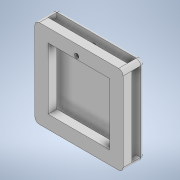
# Autodesk Inventor part: the structure
Saved by Autodesk Inventor 2022 (Build 260153000, 153)
## iProperties
Created: 2021-07-07
Part Number: the structure
Material: Generic
Document SubType Name: Modeling
Designer: fanam
Density: 1 g/cm^3
Appearance: Default
Author: fanam
Autodesk Inventor part; units mm, degrees
ref_plane "YZ Plane" through (0, 0, 0) normal (1, 0, 0) x (0, 1, 0)
ref_plane "XZ Plane" through (0, 0, 0) normal (0, 1, 0) x (-1, 0, 0)
ref_plane "XY Plane" through (0, 0, 0) normal (0, 0, 1) x (1, 0, 0)
sketch "Sketch1" plane through (0, 0, 0) normal (0, 0, 1) x (1, 0, 0)
  line L0 (0, 0) -> (1000, 0)
  line L1 (1000, 0) -> (1000, 1000)
  line L2 (1000, 1000) -> (0, 1000)
  line L3 (0, 1000) -> (0, 0)
  dimension "d0" = 1000
  dimension "d1" = 1000
  constraints: 8 end point, 2 parallel, 1 horizontal, 1 perpendicular
  measures "d0" distance of L2.end L1.end
  measures "d1" distance of L1.end L0.end
extrude "Extrusion1" add sketch "Sketch1" along normal blind 250
sketch "Sketch6" plane through (0, 1000, 0) normal (0, 1, 0) x (1, 0, 0)
  line L0 (50, -150) -> (950, -150)
  line L1 (950, -150) -> (950, -50)
  line L2 (950, -50) -> (50, -50)
  line L3 (50, -50) -> (50, -150)
  line L4 (1000, 0) -> (0, 0) projected
  line L5 (1000, 0) -> (1000, -250) projected
  dimension "d14" = 900
  dimension "d15" = 100
  dimension "d16" = 50
  dimension "d17" = 50
  constraints: 8 end point, 2 parallel, 1 horizontal, 1 perpendicular
  measures "d14" distance of L0.start L0.end
  measures "d15" distance of L0.end L1.end
  measures "d16" distance between parallel lines of L2 L4
  measures "d17" distance between parallel lines of L5 L1
extrude "Extrusion3" cut sketch "Sketch6" against normal blind 1000
sketch "Sketch7" plane through (1000, 0, 0) normal (1, 0, 0) x (0, 0, -1)
  line L0 (-150, 950) -> (-50, 950)
  line L1 (-50, 950) -> (-50, 50)
  line L2 (-50, 50) -> (-150, 50)
  line L3 (-150, 50) -> (-150, 950)
  line L4 (0, 0) -> (0, 1000) projected
  line L5 (0, 0) -> (-250, 0) projected
  dimension "d20" = 900
  dimension "d21" = 100
  dimension "d22" = 50
  dimension "d23" = 50
  constraints: 8 end point, 2 parallel, 1 horizontal, 1 perpendicular
  measures "d20" distance of L2.end L0.start
  measures "d21" distance of L1.end L2.end
  measures "d22" distance between parallel lines of L4 L1
  measures "d23" distance between parallel lines of L5 L2
extrude "Extrusion4" cut sketch "Sketch7" against normal blind 1000
sketch "Sketch8" plane through (0, 0, 250) normal (0, 0, 1) x (1, 0, 0)
  line L0 (150, 150) -> (850, 150)
  line L1 (850, 150) -> (850, 850)
  line L2 (850, 850) -> (150, 850)
  line L3 (150, 850) -> (150, 150)
  line L4 (1000, 0) -> (1000, 1000) projected
  line L5 (1000, 1000) -> (0, 1000) projected
  point P0 (0, 0)
  dimension "d26" = 700
  dimension "d27" = 700
  dimension "d28" = 150
  dimension "d29" = 150
  constraints: 8 end point, 2 parallel, 1 horizontal, 1 perpendicular
  measures "d26" distance of L1.end L2.end
  measures "d27" distance of L0.end L1.end
  measures "d28" distance between parallel lines of L4 L1
  measures "d29" distance between parallel lines of L5 L2
extrude "Extrusion5" cut sketch "Sketch8" against normal blind 125
fillet "Fillet1" radius 50 1 edges at (0, 500, 0)
fillet "Fillet2" radius 50 3 edges at (14.6446, 1000, 14.6446) (0, 1000, 149.9999) (525, 1000, 0)
fillet "Fillet3" radius 50 3 edges at (1000, 985.3554, 14.6446) (1000, 1000, 149.9999) (1000, 475, 0)
fillet "Fillet4" radius 50 5 edges at (985.3554, 0, 14.6446) (1000, 0, 149.9999) (14.6446, 0, 14.6446) (0, 0, 149.9999) (500, 0, 0)
sketch "Sketch9" plane through (0, 0, 0) normal (0, 0, -1) x (-1, 0, 0)
  point P0 (0, 0)
  point P1 (-473.9971, 885.0433)
hole "Hole1" at (473.9971, 885.0433, 0) direction (0, 0, 1) diameter 50 end through all
body "Solid1"
